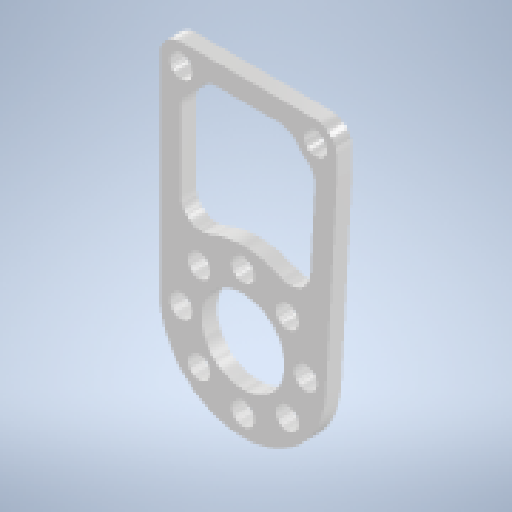
# Autodesk Inventor part: newnewude_2
Saved by Autodesk Inventor 2024 (Build 280153000, 153)
## iProperties
Created: 2024-01-04
Part Number: newnewude_2
Material: アルミニウム 2014-T4
Document SubType Name: Modeling
Designer: right
Mass: 0.943716 g
Surface Area: 7.87242 cm^2
Volume: 0.337042 cm^3
Density: 2.8 g/cm^3
Appearance: サテン
Author: right
Autodesk Inventor part; units mm, degrees
ref_plane "YZ Plane" through (0, 0, 0) normal (1, 0, 0) x (0, 1, 0)
ref_plane "XZ Plane" through (0, 0, 0) normal (0, 1, 0) x (-1, 0, 0)
ref_plane "XY Plane" through (0, 0, 0) normal (0, 0, 1) x (1, 0, 0)
sketch "スケッチ1" plane through (0, 0, 0) normal (0, 0, 1) x (1, 0, 0)
  circle A0 centre (5.6422, -7.875) radius 1 projected
  circle A1 centre (-7.3578, -7.875) radius 1 projected
  circle A2 centre (5.6422, -7.875) radius 1.1
  circle A3 centre (-7.3578, -7.875) radius 1.1
  circle A4 centre (-1.3578, -27.875) radius 4.1 projected
  circle A5 centre (-1.3578, -27.875) radius 4
  circle A6 centre (4.6422, -27.875) radius 1.1
  circle A7 centre (-1.3578, -27.875) radius 6 construction
  circle A8 centre (2.8849, -23.6324) radius 1.1
  circle A9 centre (-1.3578, -21.875) radius 1.1
  circle A10 centre (-5.6004, -23.6324) radius 1.1
  circle A11 centre (-7.3578, -27.875) radius 1.1
  circle A12 centre (-5.6004, -32.1176) radius 1.1
  circle A13 centre (-1.3578, -33.875) radius 1.1
  circle A14 centre (2.8849, -32.1176) radius 1.1
  line L0 (7.6422, -5.875) -> (-9.3578, -5.875)
  line L1 (-9.3578, -5.875) -> (-9.3578, -9.875)
  line L2 (-9.3578, -9.875) -> (7.6422, -9.875)
  line L3 (7.6422, -9.875) -> (7.6422, -5.875)
  circle A15 centre (-1.3578, -27.875) radius 8
  line L4 (6.6302, -28.3134) -> (7.6422, -9.875)
  line L5 (-9.3578, -27.875) -> (-9.3578, -9.875)
  circle A16 centre (5.6422, -7.875) radius 2
  circle A17 centre (-7.3578, -7.875) radius 2
  point P0 (0, 0)
  point P1 (5.6422, -5.875)
  point P2 (-7.3578, -5.875)
  point P3 (-9.3578, -7.875)
  point P4 (7.6422, -7.875)
  dimension "d4" = 12
  dimension "d0" = 2.2
  dimension "d1" = 2.2
  dimension "d2" = 8
  dimension "d3" = 2.2
  dimension "d7" = 360
  dimension "d9" = 16
  dimension "d10" = 4
  dimension "d11" = 4
  constraints: 14 centre point, 12 end point, 7 coincident, 6 tangent, 2 horizontal alignment, 2 parallel, 2 point on circle, 1 horizontal, 1 perpendicular, 19 other
  measures "d0" diameter of A2
  measures "d1" diameter of A3
  measures "d2" diameter of A5
  measures "d3" diameter of A6
  measures "d9" diameter of A15
  measures "d10" diameter of A16
  measures "d11" diameter of A17
extrude "押し出し1" add sketch "スケッチ1" along normal blind 1.5 contours A4 | A16 L2 A17 L0 | A16 | L3 L2 A16 | A17 | L2 L4 A15 L5 | A17 L2 L1 | A15
sketch "スケッチ2" plane through (0, 0, 1.5) normal (0, 0, 1) x (1, 0, 0)
  arc A0 (-7.3578, -5.875) -> (-9.3578, -7.875) centre (-7.3578, -7.875) ccw projected
  line L0 (-9.3578, -7.875) -> (-9.3578, -27.875) projected
  arc A1 (-9.3578, -27.875) -> (6.6302, -28.3134) centre (-1.3578, -27.875) ccw projected
  line L1 (6.6302, -28.3134) -> (7.6422, -9.875) projected
  line L2 (7.6422, -9.875) -> (7.6422, -7.875) projected
  arc A2 (7.6422, -7.875) -> (5.6422, -5.875) centre (5.6422, -7.875) ccw projected
  line L3 (5.6422, -5.875) -> (-7.3578, -5.875) projected
  circle A3 centre (4.6422, -27.875) radius 1.1 projected
  circle A4 centre (2.8849, -23.6324) radius 1.1 projected
  circle A5 centre (-1.3578, -21.875) radius 1.1 projected
  circle A6 centre (-5.6004, -23.6324) radius 1.1 projected
  circle A7 centre (-7.3578, -27.875) radius 1.1 projected
  circle A8 centre (-5.6004, -32.1176) radius 1.1 projected
  circle A9 centre (-1.3578, -33.875) radius 1.1 projected
  circle A10 centre (2.8849, -32.1176) radius 1.1 projected
  circle A11 centre (-1.3578, -27.875) radius 4 projected
  circle A12 centre (5.6422, -7.875) radius 1.1 projected
  circle A13 centre (-7.3578, -7.875) radius 1.1 projected
  line L4 (5.6422, -9.8202) -> (4.6332, -28.2038)
  arc A14 (-7.3578, -27.875) -> (4.6332, -28.2038) centre (-1.3578, -27.875) ccw
  line L5 (-7.3578, -27.875) -> (-7.3578, -7.875)
  line L6 (-7.3578, -7.875) -> (5.6422, -7.875)
  line L7 (5.6422, -7.875) -> (5.6422, -9.8202)
  circle A15 centre (5.6422, -7.875) radius 2
  circle A16 centre (-7.3578, -7.875) radius 2
  circle A17 centre (-1.3578, -27.875) radius 8
  point P0 (0, 0)
  point P1 (-7.3578, -22.5835)
  point P2 (4.9232, -22.9203)
  point P3 (5.6392, -9.875)
  point P4 (3.6422, -7.875)
  point P5 (-5.3578, -7.875)
  point P6 (-7.3578, -9.875)
  dimension "d14" = 2
  dimension "d15" = 16
  constraints: 8 end point, 4 centre point, 3 coincident, 2 point on circle, 1 concentric, 1 tangent, 4 other
  measures "d14" distance between parallel lines of L1 L4
  measures "d15" diameter of A17
extrude "押し出し2" cut sketch "スケッチ2" against normal through all contours L6 A15 L4 A17 L5 A16
fillet "フィレット1" radius 2 6 edges at (4.9232, -22.9203, 0.75) (-7.3578, -22.5835, 0.75) (-7.3578, -9.875, 0.75) (-5.3578, -7.875, 0.75) (5.6392, -9.875, 0.75) (3.6422, -7.875, 0.75)
